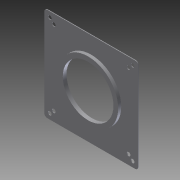
# Autodesk Inventor part: 4
Saved by Autodesk Inventor 2011 (Build 150239000, 239)
## iProperties
Created: 2011-09-17
Part Number: 4
Document SubType Name: Modeling
Designer: Matthew
Density: 1 g/cm^3
Author: Matthew
Autodesk Inventor part; units mm, degrees
ref_plane "YZ Plane" through (0, 0, 0) normal (1, 0, 0) x (0, 1, 0)
ref_plane "XZ Plane" through (0, 0, 0) normal (0, 1, 0) x (-1, 0, 0)
ref_plane "XY Plane" through (0, 0, 0) normal (0, 0, 1) x (1, 0, 0)
sketch "Sketch1" plane through (0, 0, 0) normal (0, 0, 1) x (1, 0, 0)
  line L0 (-25.4072, 25.3665) -> (76.1928, 25.3665)
  line L1 (76.1928, 25.3665) -> (76.1928, -76.2335)
  line L2 (76.1928, -76.2335) -> (-25.4072, -76.2335)
  line L3 (-25.4072, -76.2335) -> (-25.4072, 25.3665)
  point P0 (0, 0)
  dimension "d0" = 101.6
  dimension "d1" = 101.6
  constraints: 8 end point, 2 parallel, 1 horizontal, 1 perpendicular
  measures "d0" distance of L1.end L2.end
  measures "d1" distance of L0.end L1.end
extrude "Extrusion1" add sketch "Sketch1" along normal blind 0.7366
sketch "Sketch2" plane through (0, 0, 0.7366) normal (0, 0, 1) x (1, 0, 0)
  line L0 (-25.4072, 25.3665) -> (76.1928, -76.2335)
  line L1 (76.1928, 25.3665) -> (-25.4072, -76.2335)
  circle A0 centre (25.3928, -25.4335) radius 27.432
  point P0 (0, 0)
  dimension "d4" = 54.864
  constraints: 4 end point, 1 centre point, 1 midpoint, 1 perpendicular
  measures "d4" diameter of A0
extrude "Extrusion2" cut sketch "Sketch2" against normal blind 0.7366
sketch "Sketch3" plane through (0, 0, 0.7366) normal (0, 0, 1) x (1, 0, 0)
  line L0 (-25.4072, -76.2335) -> (-25.4072, 25.3665) projected
  line L1 (-25.4072, 25.3665) -> (-25.4072, -25.4335)
  line L2 (-25.4072, -25.4335) -> (-25.4072, 19.4102)
  line L3 (-25.4072, 25.3665) -> (76.1928, -76.2335)
  line L4 (76.1928, 25.3665) -> (-25.4072, -76.2335)
  circle A0 centre (-19.4509, 19.4102) radius 1.9812
  point P0 (0, 0)
  dimension "d7" = 44.8437
  dimension "d8" = 3.9624
  constraints: 8 end point, 2 point on line, 1 centre point, 1 midpoint, 1 perpendicular
  measures "d7" distance of L1.end L2.end
  measures "d8" diameter of A0
extrude "Extrusion3" cut sketch "Sketch3" against normal blind 0.7366 contours A0 L3 | L3 A0
sketch "Sketch4" plane through (0, 0, 0.7366) normal (0, 0, 1) x (1, 0, 0)
  line L0 (-25.4072, -76.2335) -> (76.1928, 25.3665)
  line L1 (-25.4072, 25.3665) -> (76.1928, -76.2335)
  circle A0 centre (70.2365, 19.4102) radius 1.9819
  circle A1 centre (70.2365, -70.2772) radius 1.983
  circle A2 centre (-19.4509, -70.2772) radius 1.9812
  point P0 (0, 0)
  constraints: 4 end point, 3 centre point, 3 point on line, 1 perpendicular
extrude "Extrusion4" cut sketch "Sketch4" against normal blind 0.7366
sketch "Sketch5" plane through (0, 0, 0.7366) normal (0, 0, 1) x (1, 0, 0)
  circle A0 centre (25.3928, -25.4335) radius 27.432 projected
  circle A1 centre (25.3928, -25.4335) radius 29.972
  circle A2 centre (25.3928, -25.4335) radius 32.512
  point P0 (0, 0)
  dimension "d13" = 59.944
  dimension "d14" = 65.024
  constraints: 2 centre point, 2 coincident
  measures "d13" diameter of A1
  measures "d14" diameter of A2
extrude "Extrusion5" add sketch "Sketch5" along normal blind 6.6548 contours A2
fillet "Fillet1" radius 3.175 4 edges at (-25.4072, 25.3665, 0.3683) (76.1928, 25.3665, 0.3683) (76.1928, -76.2335, 0.3683) (-25.4072, -76.2335, 0.3683)
sketch "Sketch6" plane through (25.3928, -25.4335, 7.3914) normal (0, 0, 1) x (1, 0, 0)
  circle A0 centre (0, 0) radius 29.972 projected
  circle A1 centre (0, 0) radius 32.512 projected
  point P0 (-25.3928, 25.4335)
extrude "Extrusion6" cut sketch "Sketch6" against normal blind 3.3274
sketch "Sketch7" plane through (25.3928, -25.4335, 0.7366) normal (0, 0, 1) x (1, 0, 0)
  circle A0 centre (0, 0) radius 29.972 projected
  circle A1 centre (0, 0) radius 27.432 projected
  point P0 (-25.3928, 25.4335)
extrude "Extrusion7" add sketch "Sketch7" along normal blind 3.3274
sketch "Sketch8" plane through (0, 0, 0.7366) normal (0, 0, 1) x (1, 0, 0)
  circle A0 centre (-19.4509, 19.4102) radius 1.9812 projected
  circle A1 centre (70.2365, -70.2772) radius 1.983 projected
  circle A2 centre (-19.4509, -70.2772) radius 1.9812 projected
  circle A3 centre (70.2365, 19.4102) radius 1.9819 projected
  line L0 (-19.4509, 19.4102) -> (70.2365, -70.2772)
  line L1 (-19.4509, -70.2772) -> (70.2365, 19.4102)
  line L2 (-25.4072, 25.3665) -> (76.1928, 25.3665)
  line L3 (76.1928, 25.3665) -> (76.1928, -76.2335)
  line L4 (76.1928, -76.2335) -> (-25.4072, -76.2335)
  line L5 (-25.4072, -76.2335) -> (-25.4072, 25.3665)
  line L6 (-25.4072, 25.3665) -> (-25.4072, -25.4335)
  line L7 (-25.4072, -25.4335) -> (-25.4072, 15.0541)
  circle A4 centre (-15.0948, 15.0541) radius 1.9812
  circle A5 centre (65.8804, 15.0541) radius 1.9816
  circle A6 centre (65.8804, -65.9211) radius 1.9817
  circle A7 centre (-15.0948, -65.9211) radius 1.9817
  point P0 (0, 0)
  dimension "d22" = 40.4876
  dimension "d23" = 3.9624
  constraints: 16 end point, 5 point on line, 4 centre point, 2 parallel, 2 perpendicular, 1 horizontal, 1 midpoint
  measures "d22" distance of L6.end L7.end
  measures "d23" diameter of A4
extrude "Extrusion8" cut sketch "Sketch8" against normal blind 3.3274 contours A5 L1 | L1 A5 | A6 L0 | L0 A6 | A7 L1 | L1 A7 | A4 L0 | L0 A4
body "Solid1"
